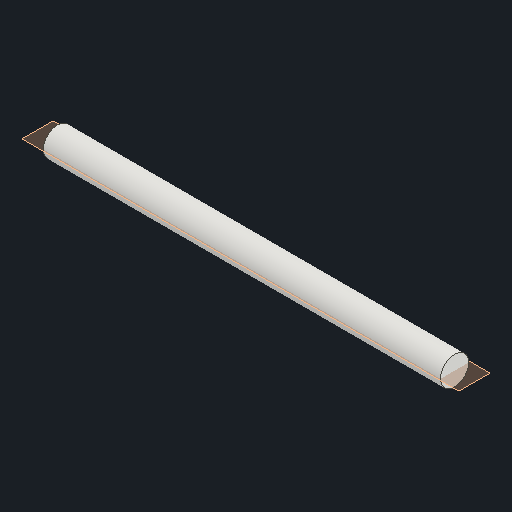
# Autodesk Inventor part: ArbreSecondaire
Saved by Autodesk Inventor 2026.2 (Build 302298010, 298A)
## iProperties
CustomPartVersion: 1
Created: 2026-03-31
Part Number: ArbreSecondaire
Material: Steel
Document SubType Name: Modeling
Designer: romai
Density: 1 g/cm^3
Appearance: Steel
Length: 350,000 mm
Author: romai
Autodesk Inventor part; units mm, degrees
ref_plane "Plan de départ" through (0, 0, 0) normal (1, 0, 0) x (0, 1, 0)
ref_plane "XY Plane" through (0, 0, 0) normal (0, 0, 1) x (1, 0, 0)
sketch "Esquisse principale" plane through (0, 0, 0) normal (0, 0, 1) x (1, 0, 0)
  line L0 (0, 0) -> (350, 0)
  line L1 (0, 0) -> (0, 12.5)
  line L2 (350, 12.5) -> (350, 0)
  line L3 (0, 12.5) -> (350, 12.5)
  dimension "d3" = 25
  constraints: 8 end point, 2 horizontal, 2 vertical
  measures "d3" diameter of L3 L0
revolve "Révolution1" add sketch "Esquisse principale" angle 360 about axis through (0, 0, 0) along (1, 0, 0)
equation "\"Length\" = 350"
